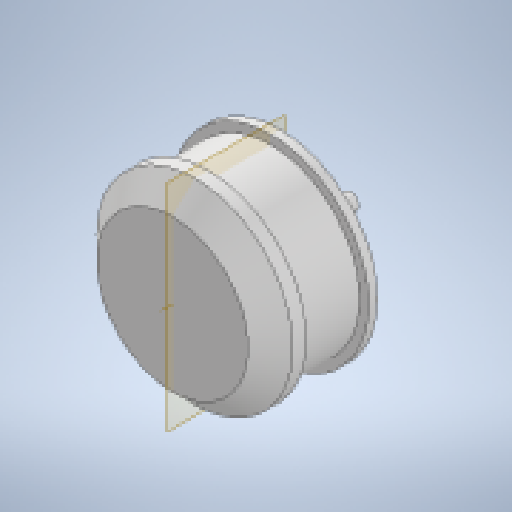
# Autodesk Inventor part: Motor
Saved by Autodesk Inventor 2025.1 (Build 291241000, 241)
## iProperties
Created: 2025-01-28
Part Number: Motor
Material: Generic
Document SubType Name: Modeling
Designer: Dimas Arif
Density: 1 g/cm^3
Appearance: Default
Author: Dimas Arif
Autodesk Inventor part; units mm, degrees
ref_plane "XZ Plane" through (0, 0, 0) normal (0, 1, 0) x (-1, 0, 0)
ref_plane "XY Plane" through (0, 0, 0) normal (0, 0, 1) x (1, 0, 0)
sketch "Sketch1" plane through (0, 0, 0) normal (0, 0, 1) x (1, 0, 0)
  circle A0 centre (-8.5, 588) radius 110
  line L0 (97.5, 88) -> (-202.5, 88) projected
  line L1 (-508.5, 482) -> (-508.5, 782) projected
  line L2 (-114.5, 1088) -> (185.5, 1088) projected
  point P0 (0, 0)
  dimension "d0" = 220
  dimension "d1" = 500
  dimension "d2" = 500
  constraints: 1 centre point
  measures "d0" diameter of A0
  measures "d1" distance from line of L1 A0.centre
  measures "d2" distance from line of L2 A0.centre
extrude "Extrusion1" add sketch "Sketch1" along normal mid plane 120
ref_plane "Work Plane1" through (-8.5, 588, 0) normal (1, 0, 0) x (0, 0, 1)
sketch "Sketch3" plane through (-8.5, 588, 0) normal (1, 0, 0) x (0, 0, 1)
  line L0 (60, -110) -> (60, 110) projected
  line L1 (-60, 110) -> (-60, -110) projected
  line L2 (-60, 110) -> (60, 110) projected
  line L3 (20, 110) -> (-50, 110)
  line L4 (-50, 110) -> (-50, 100)
  line L5 (-50, 100) -> (20, 100)
  line L6 (20, 100) -> (20, 110)
  line L7 (60, 0) -> (-58.6511, 0)
  line L8 (-84, 0) -> (84, 0) projected
  point P0 (0, 588)
  dimension "d9" = 10
  dimension "d10" = 10
  dimension "d11" = 70
  constraints: 10 end point, 2 horizontal, 2 parallel, 1 midpoint, 1 perpendicular, 1 point on line
  measures "d9" distance of L3.end L4.end
  measures "d10" distance between parallel lines of L1 L4
  measures "d11" distance of L4.end L5.end
revolve "Revolution1" cut sketch "Sketch3" angle 360 about axis through (-8.5, 588, 0) along (0, 0, 1) contours L6 L5 L4 L2
chamfer "Chamfer1" distance 25 angle 45 1 edges at (-118.5, 588, 60)
sketch "Sketch4" plane through (-8.5, 588, -60) normal (0, 0, -1) x (-1, 0, 0)
  circle A0 centre (0, 0) radius 100 construction
  circle A1 centre (0, 0) radius 85 construction
  point P0 (-8.5, -588)
  point P1 (-85, 0)
  point P2 (-42.5, -73.6122)
  point P3 (42.5, -73.6122)
  point P4 (85, 0)
  point P5 (42.5, 73.6122)
  point P6 (-42.5, 73.6122)
  dimension "d18" = 360
  constraints: 2 coincident, 1 horizontal alignment, 18 other
hole "Hole1" at (76.5, 588, -60) at (34, 514.3878, -60) at (-51, 514.3878, -60) at (-93.5, 588, -60) at (-51, 661.6122, -60) at (34, 661.6122, -60) direction (0, 0, 1) diameter 13.5 depth 10 tip angle 118 clearance for "Hex Head Cap Screw ISO 24017" size "M12" standard "ISO"
sketch "Sketch5" plane through (-8.5, 588, -60) normal (0, 0, -1) x (-1, 0, 0)
  circle A0 centre (-42.5, 73.6122) radius 6.75 projected
  circle A1 centre (42.5, 73.6122) radius 6.75 projected
  circle A2 centre (85, 0) radius 6.75 projected
  circle A3 centre (42.5, -73.6122) radius 6.75 projected
  circle A4 centre (-42.5, -73.6122) radius 6.75 projected
  circle A5 centre (-85, 0) radius 6.75 projected
  circle A6 centre (0, 0) radius 110 projected
  circle A7 centre (0, 0) radius 40
  point P0 (-8.5, -588)
  dimension "d27" = 80
  constraints: 1 centre point, 1 coincident
  measures "d27" diameter of A7
extrude "Extrusion2" add sketch "Sketch5" along normal blind 10 contours A7
sketch "Sketch6" plane through (-8.5, 588, -70) normal (0, 0, -1) x (-1, 0, 0)
  circle A0 centre (0, 0) radius 17.5
  point P0 (-8.5, -588)
  dimension "d30" = 35
  constraints: 1 centre point
  measures "d30" diameter of A0
extrude "Extrusion3" cut sketch "Sketch6" against normal up to surface (10 mm away)
sketch "Sketch7" plane through (-8.5, 588, -60) normal (0, 0, -1) x (-1, 0, 0)
  circle A0 centre (0, 0) radius 17.5 projected
  circle A1 centre (0, 0) radius 9
  point P0 (-8.5, -588)
  dimension "d33" = 18
  constraints: 1 centre point, 1 coincident
  measures "d33" diameter of A1
extrude "Extrusion4" add sketch "Sketch7" along normal blind 80 separate body contours A1
equation "\"d2\" = d1"
body "Solid1"
body "Solid2"
